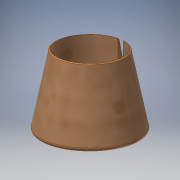
# Autodesk Inventor part: Component 43(Engine Cone)
Saved by Autodesk Inventor 2018 (Build 220112000, 112)
## iProperties
Created: 2023-04-03
Part Number: Component 43(Engine Cone)
Material: Generic
Document SubType Name: Modeling
Designer: Habib Mohamed
Density: 1 g/cm^3
Appearance: Cherry - Natural Low Gloss
Author: Habib Mohamed
Autodesk Inventor part; units mm, degrees
ref_plane "YZ Plane" through (0, 0, 0) normal (1, 0, 0) x (0, 1, 0)
ref_plane "XZ Plane" through (0, 0, 0) normal (0, 1, 0) x (-1, 0, 0)
ref_plane "XY Plane" through (0, 0, 0) normal (0, 0, 1) x (1, 0, 0)
sketch "Sketch1" plane through (0, 0, 0) normal (1, 0, 0) x (0, 1, 0)
  line L0 (11, -5) -> (11, -5.0385)
  line L1 (10.8812, -5.1853) -> (0.604, -7.3697)
  line L2 (0, -6.8807) -> (0, -6.2052)
  line L3 (0.1464, -5.8517) -> (0.8517, -5.1464)
  line L4 (1.2052, -5) -> (11, -5)
  line L5 (0, 0) -> (10.4698, 0) construction
  arc A0 (0, -6.8807) -> (0.604, -7.3697) centre (0.5, -6.8807) ccw
  arc A1 (0.1464, -5.8517) -> (0, -6.2052) centre (0.5, -6.2052) ccw
  arc A2 (10.8812, -5.1853) -> (11, -5.0385) centre (10.85, -5.0385) ccw
  arc A3 (1.2052, -5) -> (0.8517, -5.1464) centre (1.2052, -5.5) ccw
  point P0 (11, -5.16)
  point P1 (0, -7.4981)
  point P2 (0, -5.9981)
  dimension "d0" = 11
  dimension "d1" = 12
  dimension "d2" = 5.16
  dimension "d3" = 5
  dimension "d4" = 1.5
  dimension "d6" = 45
  dimension "d7" = 7.4981
  dimension "d8" = 0.5
  dimension "d9" = 0.15
  constraints: 12 end point, 8 point on circle, 8 tangent, 7 point on line, 4 centre point, 2 equal radius, 1 horizontal, 1 parallel, 1 perpendicular, 1 vertical
  measures "d0" distance from line of L5.start L0
  measures "d1" angle of L1 L4
  measures "d2" vertical distance of point (11, -5.16) L5.start
  measures "d3" vertical distance of L5.start L0.start
  measures "d4" distance of point (0, -7.498) point (0, -5.998)
  measures "d6" angle of L2 L3
  measures "d7" distance of L5.start point (0, -7.498)
  measures "d8" radius of A0
  measures "d9" radius of A2
revolve "Revolution1" add sketch "Sketch1" angle 360 about axis through (0, 0, 0) along (0, 1, 0)
sketch "Sketch2" plane through (0, 0, 0) normal (0, 1, 0) x (-1, 0, 0)
  line L0 (0.5, -6.39) -> (-0.5, -6.39)
  line L1 (-0.5, -6.39) -> (-0.5, 0)
  line L2 (-0.5, 0) -> (0.5, 0)
  line L3 (0.5, 0) -> (0.5, -6.39)
  point P0 (0, 0)
  point P1 (0, 0)
  dimension "d11" = 1
  dimension "d12" = 6.39
  constraints: 8 end point, 2 parallel, 1 coincident, 1 horizontal, 1 midpoint, 1 perpendicular
  measures "d11" distance of L1.end L2.end
  measures "d12" distance of L0.end L1.end
extrude "Extrusion1" cut sketch "Sketch2" along normal through all
body "Solid1"
